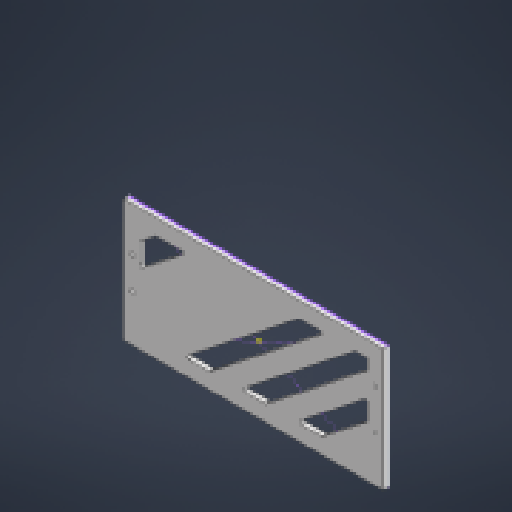
# Autodesk Inventor part: 后板2
Saved by Autodesk Inventor 2025 (Build 290162000, 162)
## iProperties
Created: 2024-12-27
Part Number: 后板2
Material: 常规
Document SubType Name: Modeling
Designer: HZD
Density: 1 g/cm^3
Appearance: 默认
Author: HZD
Autodesk Inventor part; units mm, degrees
ref_plane "YZ Plane" through (0, 0, 0) normal (1, 0, 0) x (0, 1, 0)
ref_plane "XZ Plane" through (0, 0, 0) normal (0, 1, 0) x (-1, 0, 0)
ref_plane "XY Plane" through (0, 0, 0) normal (0, 0, 1) x (1, 0, 0)
sketch "草图1" plane through (0, 0, 0) normal (0, 0, 1) x (1, 0, 0)
  line L0 (80.5, -38.1196) -> (-80.5, -38.1196)
  line L1 (-80.5, -38.1196) -> (-80.5, 38.1196)
  line L2 (-80.5, 38.1196) -> (80.5, 38.1196)
  line L3 (80.5, 38.1196) -> (80.5, -38.1196)
  line L4 (80.5, -38.1196) -> (-80.5, 38.1196) construction
  line L5 (-80.5, -38.1196) -> (80.5, 38.1196) construction
  point P0 (0, 0)
  dimension "d1" = 161
  constraints: 12 end point, 2 midpoint, 2 parallel, 1 horizontal, 1 perpendicular
  measures "d1" distance of L1.end L2.end
extrude "拉伸1" add sketch "草图1" along normal blind 3
sketch "草图2" plane through (0, 0, 3) normal (0, 0, 1) x (1, 0, 0)
  line L0 (61.6798, 137.1398) -> (-176.304, -50.1889)
  line L1 (-176.304, -50.1889) -> (-170.1188, -58.0466)
  line L2 (-170.1188, -58.0466) -> (67.865, 129.282)
  line L3 (67.865, 129.282) -> (61.6798, 137.1398)
  line L4 (80.5, 38.1196) -> (-80.5, 38.1196) projected
  line L5 (96.6798, 137.1398) -> (-141.304, -50.1889)
  line L6 (102.865, 129.282) -> (96.6798, 137.1398)
  line L7 (-135.1188, -58.0466) -> (102.865, 129.282)
  line L8 (-141.304, -50.1889) -> (-135.1188, -58.0466)
  line L9 (131.6798, 137.1398) -> (-106.304, -50.1889)
  line L10 (137.865, 129.282) -> (131.6798, 137.1398)
  line L11 (-100.1188, -58.0466) -> (137.865, 129.282)
  line L12 (-106.304, -50.1889) -> (-100.1188, -58.0466)
  line L13 (166.6798, 137.1398) -> (-71.304, -50.1889)
  line L14 (172.865, 129.282) -> (166.6798, 137.1398)
  line L15 (-65.1188, -58.0466) -> (172.865, 129.282)
  line L16 (-71.304, -50.1889) -> (-65.1188, -58.0466)
  line L17 (201.6798, 137.1398) -> (-36.304, -50.1889)
  line L18 (207.865, 129.282) -> (201.6798, 137.1398)
  line L19 (-30.1188, -58.0466) -> (207.865, 129.282)
  line L20 (-36.304, -50.1889) -> (-30.1188, -58.0466)
  line L21 (236.6798, 137.1398) -> (-1.304, -50.1889)
  line L22 (242.865, 129.282) -> (236.6798, 137.1398)
  line L23 (4.8812, -58.0466) -> (242.865, 129.282)
  line L24 (-1.304, -50.1889) -> (4.8812, -58.0466)
  line L25 (271.6798, 137.1398) -> (33.696, -50.1889)
  line L26 (277.865, 129.282) -> (271.6798, 137.1398)
  line L27 (39.8812, -58.0466) -> (277.865, 129.282)
  line L28 (33.696, -50.1889) -> (39.8812, -58.0466)
  line L29 (-80.5, 38.1196) -> (-80.5, -38.1196) projected
  line L30 (80.5, -38.1196) -> (80.5, 38.1196) projected
  line L31 (-80.5, -38.1196) -> (80.5, -38.1196) projected
  line L32 (-70.5, 28.1196) -> (70.5, 28.1196)
  line L33 (70.5, 28.1196) -> (70.5, -28.1196)
  line L34 (70.5, -28.1196) -> (-70.5, -28.1196)
  line L35 (-70.5, -28.1196) -> (-70.5, 28.1196)
  point P0 (0, 0)
  point P1 (-51.1269, 35.6177)
  point P2 (-16.1269, 35.6177)
  point P3 (18.8731, 35.6177)
  point P4 (53.8731, 35.6177)
  point P5 (88.8731, 35.6177)
  point P6 (123.8731, 35.6177)
  point P7 (158.8731, 35.6177)
  point P8 (26.733, -28.1196)
  point P9 (42.9006, -28.1196)
  point P10 (70.5, -6.3948)
  point P11 (70.5, 6.3315)
  point P12 (-8.267, -28.1196)
  point P13 (7.9006, -28.1196)
  point P14 (70.5, 21.1554)
  point P15 (63.1798, 28.1196)
  point P16 (-43.267, -28.1196)
  point P17 (-27.0994, -28.1196)
  point P18 (44.3475, 28.1196)
  point P19 (28.1798, 28.1196)
  point P20 (-70.5, -7.182)
  point P21 (-70.5, -22.0058)
  point P22 (-6.8202, 28.1196)
  point P23 (-25.6525, 28.1196)
  point P24 (-70.5, 20.3682)
  point P25 (-70.5, 5.5444)
  point P26 (-41.8202, 28.1196)
  point P27 (-60.6525, 28.1196)
  dimension "d5" = 10
  dimension "d8" = 35
  dimension "d13" = 10
  constraints: 64 end point, 2 parallel, 1 horizontal, 1 midpoint, 1 perpendicular, 57 other
  measures "d5" distance from line of L0 point (-51.127, 35.618)
  measures "d8" distance of L0.start L5.start
  measures "d13" distance between parallel lines of L4 L32
extrude "拉伸2" cut sketch "草图2" against normal blind 10 contours L32 L5 L35 L2 | L32 L15 L34 L13 | L32 L33 L19 L34 L17 | L21 L33 L23 L34
fillet "圆角1" radius 1 14 edges at (28.1798, 28.1196, 1.5) (44.3475, 28.1196, 1.5) (63.1798, 28.1196, 1.5) (70.5, 21.1554, 1.5) (70.5, 6.3315, 1.5) (26.733, -28.1196, 1.5) (42.9006, -28.1196, 1.5) (70.5, -6.3948, 1.5) (-8.267, -28.1196, 1.5) (7.9006, -28.1196, 1.5) (-43.267, -28.1196, 1.5) (-27.0994, -28.1196, 1.5) (-70.5, 5.5444, 1.5) (-41.8202, 28.1196, 1.5)
sketch "草图3" plane through (0, 0, 3) normal (0, 0, 1) x (1, 0, 0)
  ellipse E0 centre (75.5, 15.3081) end of major axis (76.7, 15.3081) minor radius 1.1476 projected
  circle A0 centre (75.5, -9.3544) radius 1.2 projected
  circle A1 centre (-75.5, 10.6456) radius 1.2 projected
  circle A2 centre (-75.5, -9.3544) radius 1.2 projected
  point P0 (0, 0)
extrude "拉伸3" cut sketch "草图3" against normal blind 10
equation "\"d14\" = d5"
equation "\"d17\" = d5"
